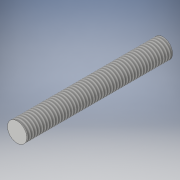
# Autodesk Inventor part: Weight_Thread_3mm
Saved by Autodesk Inventor 2019 (Build 230136000, 136)
## iProperties
Created: 2019-04-25
Part Number: Weight_Thread_3mm
Material: Generic
Document SubType Name: Modeling
Designer: 19879326
Density: 1 g/cm^3
Appearance: Default
Author: 19879326
Autodesk Inventor part; units mm, degrees
ref_plane "YZ Plane" through (0, 0, 0) normal (1, 0, 0) x (0, 1, 0)
ref_plane "XZ Plane" through (0, 0, 0) normal (0, 1, 0) x (-1, 0, 0)
ref_plane "XY Plane" through (0, 0, 0) normal (0, 0, 1) x (1, 0, 0)
sketch "Sketch1" plane through (0, 0, 0) normal (0, 0, 1) x (1, 0, 0)
  circle A0 centre (0, 0) radius 4
  dimension "d0" = 8
  constraints: 1 centre point, 1 coincident
  measures "d0" diameter of A0
extrude "Extrusion1" add sketch "Sketch1" along normal blind 60
thread "Thread1" size "M8x1.25" class "6g" standard "ANSI Metric M Profile" full length
body "Solid1"
